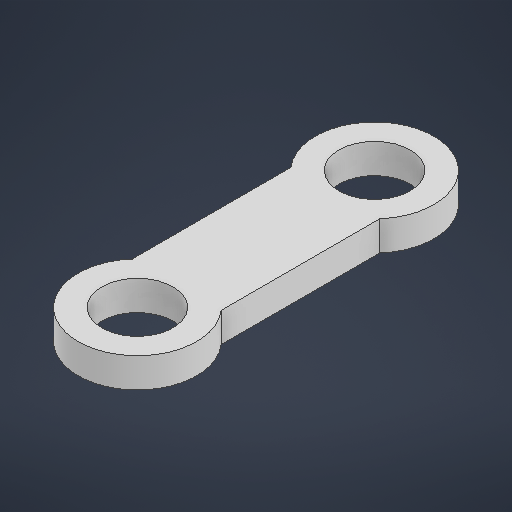
# Autodesk Inventor part: link-8-1pin
Saved by Autodesk Inventor 2025.4 (Build 294407000, 407)
## iProperties
Created: 2026-09-15
Part Number: link-8-1pin
Material: Generic
Document SubType Name: Modeling
Designer: User
Density: 1 g/cm^3
Appearance: Default
Author: User
Autodesk Inventor part; units mm, degrees
ref_plane "YZ Plane" through (0, 0, 0) normal (1, 0, 0) x (0, 1, 0)
ref_plane "XZ Plane" through (0, 0, 0) normal (0, 1, 0) x (-1, 0, 0)
sketch "Sketch1" plane through (0, 0, 0) normal (0, 1, 0) x (-1, 0, 0)
  line L0 (-1.5, -4) -> (1.5, -4)
  line L1 (1.5, -4) -> (1.5, 4)
  line L2 (1.5, 4) -> (-1.5, 4)
  line L3 (-1.5, 4) -> (-1.5, -4)
  line L4 (-1.5, -4) -> (1.5, 4) construction
  line L5 (1.5, -4) -> (-1.5, 4) construction
  circle A0 centre (0, 4) radius 1.2
  circle A1 centre (0, -4) radius 1.2
  circle A2 centre (0, -4) radius 2
  circle A3 centre (0, 4) radius 2
  point P0 (0, 0)
  point P1 (-1.5, -2.6771)
  point P2 (1.5, -2.6771)
  point P3 (1.5, 2.6771)
  point P4 (-1.5, 2.6771)
  dimension "d0" = 3
  dimension "linkPitch" = 8
  dimension "d2" = 2.4
  dimension "d3" = 2.4
  dimension "d4" = 4
  dimension "d5" = 4
  constraints: 12 end point, 4 centre point, 4 midpoint, 2 coincident, 2 parallel, 1 horizontal, 1 perpendicular
  measures "d0" distance of L2.end L1.end
  measures "linkPitch" distance of L1.end L0.end
  measures "d2" diameter of A0
  measures "d3" diameter of A1
  measures "d4" diameter of A2
  measures "d5" diameter of A3
extrude "Extrusion1" add sketch "Sketch1" along normal blind 1 contours A1 L0 L3 A2 L1 | L0 L1 A2 L3 A1 | A2 L3 A3 L1 | A3 L3 L2 A0 L1 | L1 L2 A0 L3 A3
ref_plane "Work Plane1" through (0, 0.5, 0) normal (0, 1, 0) x (1, 0, 0)
sketch "Sketch2" plane through (0, 1, 0) normal (0, 1, 0) x (1, 0, 0)
  line L0 (-1.5, 2.6771) -> (-1.5, -2.6771) projected
  arc A0 (-1.5, -2.6771) -> (1.5, -2.6771) centre (0, -4) ccw projected
  line L1 (1.5, -2.6771) -> (1.5, 2.6771) projected
  arc A1 (1.5, 2.6771) -> (-1.5, 2.6771) centre (0, 4) ccw projected
  circle A2 centre (0, 4) radius 1.2 projected
  circle A3 centre (0, -4) radius 1.2 projected
  circle A4 centre (0, -4) radius 1
  point P0 (0, 0)
  dimension "d17" = 2
  constraints: 1 centre point, 1 coincident
  measures "d17" diameter of A4
extrude "Extrusion2" [suppressed]
sketch "Sketch3" plane through (0, 1, 0) normal (0, 1, 0) x (1, 0, 0)
  line L0 (-1.5, 2.6771) -> (-1.5, -2.6771) projected
  arc A0 (-1.5, -2.6771) -> (1.5, -2.6771) centre (0, -4) ccw projected
  line L1 (1.5, -2.6771) -> (1.5, 2.6771) projected
  arc A1 (1.5, 2.6771) -> (-1.5, 2.6771) centre (0, 4) ccw projected
  circle A2 centre (0, 4) radius 1.2 projected
  circle A3 centre (0, -4) radius 1.2 projected
  circle A4 centre (0, 4) radius 1
  point P0 (0, 0)
  dimension "d18" = 2
  constraints: 1 centre point, 1 coincident
  measures "d18" diameter of A4
extrude "Extrusion3" [suppressed]
sketch "Sketch4" plane through (0, 1, 0) normal (0, 1, 0) x (1, 0, 0)
  line L0 (-1.5, 2.6771) -> (-1.5, -2.6771) projected
  arc A0 (-1.5, -2.6771) -> (1.5, -2.6771) centre (0, -4) ccw projected
  line L1 (1.5, -2.6771) -> (1.5, 2.6771) projected
  arc A1 (1.5, 2.6771) -> (-1.5, 2.6771) centre (0, 4) ccw projected
  circle A2 centre (0, 4) radius 1.2 projected
  circle A3 centre (0, -4) radius 1.2 projected
  point P0 (0, 0)
extrude "Extrusion4" [suppressed]
sketch "Sketch5" plane through (0, 1, 0) normal (0, 1, 0) x (1, 0, 0)
  line L0 (-1.5, 2.6771) -> (-1.5, -2.6771) projected
  arc A0 (-1.5, -2.6771) -> (1.5, -2.6771) centre (0, -4) ccw projected
  line L1 (1.5, -2.6771) -> (1.5, 2.6771) projected
  arc A1 (1.5, 2.6771) -> (-1.5, 2.6771) centre (0, 4) ccw projected
  circle A2 centre (0, 4) radius 1.2 projected
  point P0 (0, 0)
extrude "Extrusion5" [suppressed]
equation "\"d2\" = d3"
equation "\"d5\" = d4"
body "Solid1"
